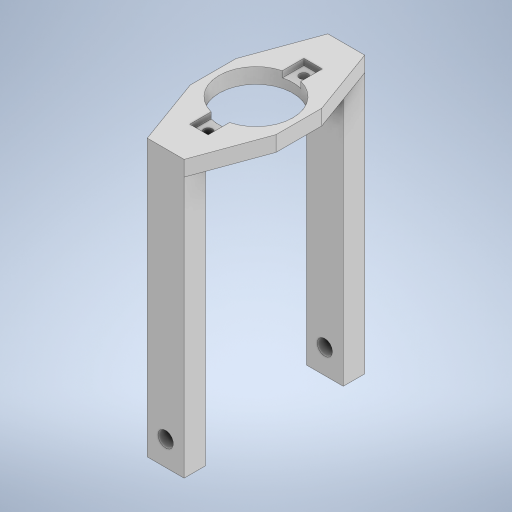
# Autodesk Inventor part: m500 hires mount
Saved by Autodesk Inventor 2023 (Build 270158000, 158)
## iProperties
Created: 2022-08-11
Part Number: m500 hires mount
Material: Generic
Document SubType Name: Modeling
Designer: Eli
Density: 1 g/cm^3
Appearance: Default
Author: Eli
Autodesk Inventor part; units mm, degrees
ref_plane "YZ Plane" through (0, 0, 0) normal (1, 0, 0) x (0, 1, 0)
ref_plane "XZ Plane" through (0, 0, 0) normal (0, 1, 0) x (-1, 0, 0)
ref_plane "XY Plane" through (0, 0, 0) normal (0, 0, 1) x (1, 0, 0)
sketch "Sketch1" plane through (0, 0, 0) normal (0, 1, 0) x (-1, 0, 0)
  line L0 (0, 0) -> (-17.78, 0)
  line L1 (-17.78, 0) -> (-17.78, -37.3888)
  line L2 (-17.78, -37.3888) -> (0, -37.3888)
  line L3 (0, -37.3888) -> (0, 0)
  circle A0 centre (-8.89, -18.6944) radius 7.62
  line L4 (0, -18.6944) -> (-17.78, -18.6944) construction
  line L5 (-8.89, -37.3888) -> (-8.89, 0) construction
  circle A1 centre (-8.89, -28.6004) radius 0.889
  circle A2 centre (-8.89, -8.7884) radius 0.889
  dimension "d0" = 37.3888
  dimension "d1" = 17.78
  dimension "d2" = 15.24
  dimension "d3" = 1.778
  dimension "d4" = 19.812
  constraints: 12 end point, 5 midpoint, 3 centre point, 2 parallel, 2 point on line, 1 equal radius, 1 horizontal, 1 perpendicular, 1 symmetric about line
  measures "d0" distance of L2.end L0.start
  measures "d1" distance of L1.end L2.end
  measures "d2" diameter of A0
  measures "d3" diameter of A1
  measures "d4" distance of A1.centre A2.centre
extrude "Extrusion1" add sketch "Sketch1" along normal blind 3.175
sketch "Sketch2" plane through (0, 3.175, 0) normal (0, 1, 0) x (1, 0, 0)
  line L0 (6.985, 6.8834) -> (10.795, 6.8834)
  line L1 (10.795, 6.8834) -> (10.795, 12.3482)
  line L2 (10.795, 12.3482) -> (6.985, 12.3482)
  line L3 (6.985, 12.3482) -> (6.985, 6.8834)
  circle A0 centre (8.89, 8.7884) radius 0.889 construction
  line L4 (8.89, 8.7884) -> (8.001, 8.7884) construction
  line L5 (8.89, 8.7884) -> (8.89, 9.6774) construction
  line L6 (6.985, 25.0482) -> (10.795, 25.0482)
  line L7 (10.795, 25.0482) -> (10.795, 30.513)
  line L8 (10.795, 30.513) -> (6.985, 30.513)
  line L9 (6.985, 30.513) -> (6.985, 25.0482)
  circle A1 centre (8.89, 28.6004) radius 0.889 construction
  line L10 (8.001, 28.6004) -> (8.89, 28.6004) construction
  point P0 (0, 0)
  point P1 (8.4455, 8.7884)
  point P2 (8.4455, 28.6004)
  dimension "d8" = 3.81
  dimension "d11" = 1.905
  dimension "d12" = 1.9126
  dimension "d13" = 12.7
  constraints: 22 end point, 4 horizontal, 4 parallel, 3 perpendicular, 2 equal length, 2 midpoint, 2 point on circle, 1 collinear, 1 horizontal alignment, 2 other
  measures "d8" distance of L1.end L2.end
  measures "d11" distance from line of point (8.445, 8.788) L0
  measures "d12" distance from line of L8 point (8.445, 28.6)
  measures "d13" distance between parallel lines of L2 L6
extrude "Extrusion2" cut sketch "Sketch2" against normal blind 1.27
sketch "Sketch3" plane through (0, 3.175, 0) normal (0, 1, 0) x (1, 0, 0)
  line L0 (17.78, 37.3888) -> (0, 37.3888) projected
  line L1 (12.7, 37.3888) -> (5.08, 37.3888)
  line L2 (5.08, 37.3888) -> (5.08, 32.9438)
  line L3 (5.08, 32.9438) -> (12.7, 32.9438)
  line L4 (12.7, 32.9438) -> (12.7, 37.3888)
  line L5 (0, 0) -> (17.78, 0) projected
  line L6 (12.7, 0) -> (5.08, 0)
  line L7 (5.08, 0) -> (5.08, 4.445)
  line L8 (5.08, 4.445) -> (12.7, 4.445)
  line L9 (12.7, 4.445) -> (12.7, 0)
  line L10 (17.78, 0) -> (17.78, 37.3888) construction
  line L11 (17.78, 18.6944) -> (0, 18.6944) construction
  line L12 (0, 37.3888) -> (0, 0) construction
  circle A0 centre (8.89, 18.6944) radius 7.62 construction
  line L13 (8.89, 18.6944) -> (8.89, 11.0744) construction
  point P0 (8.89, 4.445)
  point P1 (5.08, 37.3888)
  dimension "d14" = 28.4988
  dimension "d15" = 7.62
  constraints: 20 end point, 5 parallel, 3 midpoint, 2 horizontal, 2 perpendicular, 2 point on line, 1 collinear, 1 vertical, 1 vertical alignment, 3 other
  measures "d14" distance from line of point (8.89, 4.445) L3
  measures "d15" distance between parallel lines of L7 L9
extrude "Extrusion3" add sketch "Sketch3" against normal blind 57.15
sketch "Sketch4" plane through (17.78, 3.175, -37.3888) normal (0, 0, -1) x (-1, 0, 0)
  line L0 (12.7, -57.15) -> (5.08, -57.15) projected
  line L1 (12.7, -3.175) -> (12.7, -57.15) projected
  point P0 (17.78, -3.175)
  point P1 (8.89, -52.07)
  dimension "d18" = 5.08
  dimension "d19" = 3.81
  measures "d18" distance from line of L0 point (8.89, -52.07)
  measures "d19" distance from line of L1 point (8.89, -52.07)
hole "Hole1" at (8.89, -48.895, -37.3888) direction (0, 0, 1) diameter 3.175 depth 37.3888
chamfer "Chamfer1" distance 5.08 angle 70 1 edges at (17.78, 1.5875, -37.3888) measured on face at (8.89, -15.7692, -37.3888)
chamfer "Chamfer2" distance 5.08 angle 70 1 edges at (0, 1.5875, -37.3888) measured on face at (8.89, -15.7692, -37.3888)
chamfer "Chamfer3" distance 5.08 angle 70 1 edges at (17.78, 1.5875, 0) measured on face at (8.89, -15.7692, 0)
chamfer "Chamfer4" distance 5.08 angle 70 1 edges at (0, 1.5875, 0) measured on face at (8.89, -15.7692, 0)
body "Solid1"
